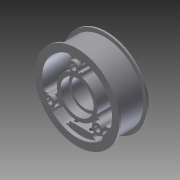
# Autodesk Inventor part: wheel 3in custom
Saved by Autodesk Inventor 2012 (Build 160160000, 160)
## iProperties
Created: 2013-08-02
Part Number: wheel 3in custom
Material: Default
Document SubType Name: Modeling
Designer: Bryce
Density: 1 g/cm^3
Author: Bryce
Autodesk Inventor part; units mm, degrees
ref_plane "YZ Plane" through (0, 0, 0) normal (1, 0, 0) x (0, 1, 0)
ref_plane "XZ Plane" through (0, 0, 0) normal (0, 1, 0) x (-1, 0, 0)
ref_plane "XY Plane" through (0, 0, 0) normal (0, 0, 1) x (1, 0, 0)
sketch "Sketch1" plane through (0, 0, 0) normal (0, 0, 1) x (1, 0, 0)
  circle A0 centre (0, 0) radius 36.5125
  circle A1 centre (0, 0) radius 33.3375
  circle A2 centre (0, 23.8125) radius 2.286
  circle A3 centre (0, 0) radius 14.2875
  line L0 (0, 0) -> (0, 23.8125) construction
  line L1 (3.175, 17.1714) -> (3.175, 20.2627)
  line L2 (3.175, 27.3623) -> (3.175, 29.9949)
  arc A4 (16.4584, -5.8361) -> (3.175, 17.1714) centre (0, 0) ccw
  arc A5 (3.175, 20.2627) -> (3.175, 27.3623) centre (0, 23.8125) ccw
  arc A6 (27.5639, -12.2478) -> (3.175, 29.9949) centre (0, 0) ccw
  line L3 (0, 0) -> (20.6222, -11.9062) construction
  line L4 (16.4584, -5.8361) -> (19.1355, -7.3817)
  line L5 (25.2839, -10.9315) -> (27.5639, -12.2478)
  arc A7 (25.2839, -10.9315) -> (19.1355, -7.3817) centre (20.6222, -11.9062) ccw
  circle A8 centre (0, 0) radius 11.9062
  circle A9 centre (-20.6222, -11.9062) radius 2.286
  line L6 (-16.4584, -5.8361) -> (-19.1355, -7.3817)
  line L7 (-25.2839, -10.9315) -> (-27.5639, -12.2478)
  arc A10 (-3.175, 17.1714) -> (-16.4584, -5.8361) centre (0, 0) ccw
  arc A11 (-19.1355, -7.3817) -> (-25.2839, -10.9315) centre (-20.6222, -11.9062) ccw
  arc A12 (-3.175, 29.9949) -> (-27.5639, -12.2478) centre (0, 0) ccw
  line L8 (0, 0) -> (0, 23.8125) construction
  line L9 (-3.175, 17.1714) -> (-3.175, 20.2627)
  line L10 (-3.175, 27.3623) -> (-3.175, 29.9949)
  arc A13 (-3.175, 27.3623) -> (-3.175, 20.2627) centre (0, 23.8125) ccw
  circle A14 centre (20.6222, -11.9063) radius 2.286
  line L11 (13.2834, -11.3353) -> (15.9605, -12.881)
  line L12 (22.1089, -16.4308) -> (24.3889, -17.7471)
  arc A15 (-13.2834, -11.3353) -> (13.2834, -11.3353) centre (0, 0) ccw
  arc A16 (15.9605, -12.881) -> (22.1089, -16.4308) centre (20.6222, -11.9063) ccw
  arc A17 (-24.3889, -17.7471) -> (24.3889, -17.7471) centre (0, 0) ccw
  line L13 (0, 0) -> (-20.6222, -11.9062) construction
  line L14 (-13.2834, -11.3353) -> (-15.9605, -12.881)
  line L15 (-22.1089, -16.4308) -> (-24.3889, -17.7471)
  arc A18 (-22.1089, -16.4308) -> (-15.9605, -12.881) centre (-20.6222, -11.9062) ccw
  line L16 (9.525, -28.6191) -> (9.525, -23.8566) construction
  line L17 (9.525, -23.8566) -> (-9.525, -23.8566)
  line L18 (-9.525, -23.8566) -> (-9.525, -28.6191) construction
  arc A19 (-14.1938, -26.6142) -> (-9.525, -23.8566) centre (-12.6997, -23.8127) ccw
  arc A20 (9.525, -23.8566) -> (14.1938, -26.6142) centre (12.6997, -23.8127) ccw
  dimension "d0" = 73.025
  dimension "d1" = 66.675
  dimension "d8" = 4.572
  dimension "d10" = 23.8125
  dimension "d11" = 28.575
  dimension "d12" = 3.175
  dimension "d13" = 4.7625
  dimension "d14" = 17.4625
  dimension "d15" = 30.1625
  dimension "d16" = 3.175
  dimension "d17" = 4.7625
  dimension "d18" = 23.8125
  dimension "d19" = 120
  dimension "d31" = 23.8125
  dimension "d45" = 360
  dimension "d50" = 19.05
  dimension "d51" = 4.7625
  dimension "d72" = 3.175
  constraints: 38 end point, 33 point on circle, 21 centre point, 14 coincident, 4 collinear, 4 parallel, 2 tangent, 1 equal radius, 1 horizontal, 1 perpendicular, 1 vertical, 1 vertical alignment, 73 other
  measures "d0" diameter of A0
  measures "d1" diameter of A1
  measures "d8" diameter of A2
  measures "d10" distance of L0.start L0.end
  measures "d11" diameter of A3
  measures "d12" distance between parallel lines of L0 L1
  measures "d13" radius of A5
  measures "d14" radius of A4
  measures "d15" radius of A6
  measures "d16" distance between parallel lines of L3 L4
  measures "d17" radius of A7
  measures "d18" distance of L3.start L3.end
  measures "d19" angle of L3 L0
  measures "d31" diameter of A8
  measures "d50" distance of L16.end L17.end
  measures "d51" distance of L17.end L18.end
  measures "d72" radius of A19
extrude "Extrusion1" add sketch "Sketch1" along normal blind 25.4 contours A0 | A1
extrude "Extrusion2" cut sketch "Sketch1" along normal blind 23.8125 contours A0
extrude "Extrusion3" add sketch "Sketch1" along normal blind 1.5875 contours A0
fillet "Fillet1" radius 3.175 24 edges at (3.175, 20.2627, 12.7) (3.175, 27.3623, 12.7) (27.5639, -12.2478, 12.7) (25.2839, -10.9315, 12.7) (19.1355, -7.3817, 12.7) (16.4584, -5.8361, 12.7) (-3.175, 29.9949, 12.7) (-3.175, 27.3623, 12.7) (-3.175, 20.2627, 12.7) (-3.175, 17.1714, 12.7) (-16.4584, -5.8361, 12.7) (-19.1355, -7.3817, 12.7) (-25.2839, -10.9315, 12.7) (13.2834, -11.3353, 12.7) (-13.2834, -11.3353, 12.7) (15.9605, -12.881, 12.7) (-15.9605, -12.881, 12.7) (-27.5639, -12.2478, 12.7) (22.1089, -16.4308, 12.7) (-22.1089, -16.4308, 12.7) (24.3889, -17.7471, 12.7) (-24.3889, -17.7471, 12.7) (3.175, 17.1714, 12.7) (3.175, 29.9949, 12.7)
extrude "Extrusion4" add sketch "Sketch1" along normal blind 18.415 contours A3
extrude "Extrusion5" cut sketch "Sketch1" along normal blind 6.985 contours A3
sketch "Sketch2" plane through (0, 0, 25.4) normal (0, 0, 1) x (1, 0, 0)
  arc A0 (-4.5987, 25.0508) -> (-8.5662, 28.9205) centre (-7.6645, 25.8763) ccw projected
  circle A1 centre (-20.6222, -11.9062) radius 2.286 projected
  arc A2 (-11.4822, -13.1567) -> (-16.3908, -14.0918) centre (-13.5699, -15.5488) ccw projected
  arc A3 (-19.3952, -16.508) -> (-16.3908, -14.0918) centre (-20.6222, -11.9062) ccw projected
  arc A4 (-19.3952, -16.508) -> (-20.7628, -21.8788) centre (-18.5772, -19.5758) ccw projected
  arc A5 (-29.329, -7.0417) -> (-23.9939, -8.5428) centre (-26.2417, -6.3005) ccw projected
  arc A6 (-20.3992, -7.149) -> (-23.9939, -8.5428) centre (-20.6222, -11.9062) ccw projected
  arc A7 (-20.3992, -7.149) -> (-17.1351, -3.3655) centre (-20.2506, -3.9775) ccw projected
  circle A8 centre (20.6222, -11.9063) radius 2.286 projected
  arc A9 (16.3908, -14.0918) -> (19.3952, -16.508) centre (20.6222, -11.9063) ccw projected
  arc A10 (20.7628, -21.8788) -> (19.3952, -16.508) centre (18.5772, -19.5758) ccw projected
  arc A11 (23.9939, -8.5428) -> (29.329, -7.0417) centre (26.2417, -6.3005) ccw projected
  arc A12 (23.9939, -8.5428) -> (20.3992, -7.149) centre (20.6222, -11.9062) ccw projected
  arc A13 (17.1351, -3.3655) -> (20.3992, -7.149) centre (20.2506, -3.9775) ccw projected
  arc A14 (-23.9939, -8.5428) -> (-19.3952, -16.508) centre (-20.6222, -11.9062) ccw
  arc A15 (19.3952, -16.508) -> (23.9939, -8.5428) centre (20.6222, -11.9062) ccw
  arc A16 (-18.6902, -7.5532) -> (-20.3992, -7.149) centre (-20.6222, -11.9062) ccw
  arc A17 (-16.3908, -14.0918) -> (-15.8864, -12.4096) centre (-20.6222, -11.9062) ccw
  arc A18 (15.8864, -12.4096) -> (16.3908, -14.0918) centre (20.6222, -11.9062) ccw
  arc A19 (20.3992, -7.149) -> (18.6902, -7.5532) centre (20.6222, -11.9062) ccw
  circle A20 centre (0, 23.8125) radius 4.7625
  circle A21 centre (-20.6222, -11.9062) radius 4.7625
  circle A22 centre (20.6222, -11.9062) radius 4.7625
  arc A23 (16.3908, -14.0918) -> (11.4822, -13.1567) centre (13.5699, -15.5488) ccw projected
  arc A24 (17.1351, -3.3655) -> (5.6529, 16.5222) centre (0, 0) ccw projected
  arc A25 (4.0084, 21.2407) -> (5.6529, 16.5222) centre (6.6807, 19.5263) ccw projected
  arc A26 (-5.6529, 16.5222) -> (-4.0084, 21.2407) centre (-6.6807, 19.5263) ccw projected
  circle A27 centre (0, 23.8125) radius 2.286 projected
  arc A28 (4.0084, 21.2407) -> (4.5987, 25.0508) centre (0, 23.8125) ccw projected
  arc A29 (-4.5987, 25.0508) -> (-4.0084, 21.2407) centre (0, 23.8125) ccw projected
  constraints: 12 point on circle, 9 coincident, 6 centre point, 9 other
extrude "Extrusion8" add sketch "Sketch2" along normal blind 3.175
extrude "Extrusion9" add sketch "Sketch1" along normal blind 22.225 contours A17 A19 L17 A20
extrude "Extrusion10" cut sketch "Sketch1" along normal blind 3.175 contours L11 A16 L12 A17 A20 L17 A19 L15 A18 L14 A15
sketch "Sketch4" plane through (-9.525, -23.8566, 22.225) normal (0, 1, 0) x (1, 0, 0)
  line L0 (0, 0) -> (19.05, 0) projected
  circle A0 centre (3.175, 15.875) radius 1.7526
  circle A1 centre (15.875, 15.875) radius 1.7526
  circle A2 centre (3.175, 3.175) radius 1.7526
  circle A3 centre (15.875, 3.175) radius 1.7526
  line L1 (0, 22.225) -> (0, 0) projected
  line L2 (19.05, 22.225) -> (19.05, 0) projected
  line L3 (19.05, 22.225) -> (0, 22.225) projected
  dimension "d56" = 3.5052
  dimension "d59" = 3.175
  dimension "d73" = 6.35
  dimension "d74" = 3.175
  dimension "d75" = 3.175
  constraints: 4 centre point, 3 equal radius, 2 horizontal alignment, 2 vertical alignment
  measures "d56" diameter of A1
  measures "d59" distance from line of L0 A3.centre
  measures "d73" distance from line of L3 A0.centre
  measures "d74" distance from line of L1 A0.centre
  measures "d75" distance from line of L2 A1.centre
extrude "Extrusion11" cut sketch "Sketch4" against normal through all contours A0 | A1 | A2 | A3
thread "Thread1" size "6-32 UNC" class "2B" standard "ANSI Unified Screw Threads" full length
thread "Thread2" size "6-32 UNC" class "2B" standard "ANSI Unified Screw Threads" full length
thread "Thread3" size "6-32 UNC" class "2B" standard "ANSI Unified Screw Threads" full length
thread "Thread4" size "6-32 UNC" class "2B" standard "ANSI Unified Screw Threads" full length
extrude "Extrusion12" cut sketch "Sketch1" along normal blind 3.175 contours A17 A19 L17 A20
equation "\"d16\" = d12"
equation "\"d17\" = d13"
equation "\"d18\" = d10"
body "Solid1"
